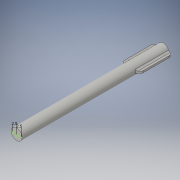
# Autodesk Inventor part: Nathan_Practice_9
Saved by Autodesk Inventor 2016 (Build 200138000, 138)
## iProperties
Created: 2017-03-09
Part Number: Nathan_Practice_9
Material: Generic
Document SubType Name: Modeling
Designer: Student
Density: 1 g/cm^3
Appearance: Default
Author: Student
Autodesk Inventor part; units mm, degrees
ref_plane "YZ Plane" through (0, 0, 0) normal (1, 0, 0) x (0, 1, 0)
ref_plane "XZ Plane" through (0, 0, 0) normal (0, 1, 0) x (-1, 0, 0)
ref_plane "XY Plane" through (0, 0, 0) normal (0, 0, 1) x (1, 0, 0)
sketch "Sketch1" plane through (0, 0, 0) normal (0, 0, 1) x (1, 0, 0)
  circle A0 centre (0, 0) radius 3
  dimension "d0" = 6
  constraints: 1 centre point, 1 coincident
  measures "d0" diameter of A0
extrude "Extrusion1" add sketch "Sketch1" along normal blind 80
sketch "Sketch2" plane through (0, 0, 0) normal (0, 1, 0) x (-1, 0, 0)
  line L0 (-3, 0) -> (3, 0) projected
  line L1 (5, 0) -> (5, 18)
  line L2 (-5, 0) -> (-5, 18)
  line L3 (-3, 0) -> (-3, 80) projected
  line L4 (3, 0) -> (3, 80) projected
  line L5 (5, 18) -> (2, 18)
  line L6 (2, 18) -> (2, 0)
  line L7 (5, 0) -> (2, 0)
  line L8 (-5, 18) -> (-2, 18)
  line L9 (-2, 18) -> (-2, 0)
  line L10 (-2, 0) -> (-5, 0)
  point P0 (0, 0)
  dimension "d3" = 2
  dimension "d4" = 2
  dimension "d6" = 18
  dimension "d9" = 3
  dimension "d10" = 18
  dimension "d11" = 3
  constraints: 16 end point, 3 perpendicular, 2 horizontal, 2 point on line, 2 vertical, 1 collinear
  measures "d3" distance of L0.start L2.start
  measures "d4" distance of L0.end L1.start
  measures "d6" distance of L2.start L2.end
  measures "d9" distance of L1.end L5.end
  measures "d10" distance between parallel lines of L5 L7
  measures "d11" distance of L2.end L8.end
extrude "Extrusion2" add sketch "Sketch2" along normal mid plane 1
fillet "Fillet1" radius 2 4 edges at (5, 0, 18) (-5, 0, 18) (-5, 0, 0) (5, 0, 0)
fillet "Fillet2" radius 1 4 edges at (-2.958, 0.5, 9) (-2.958, -0.5, 9) (2.958, -0.5, 9) (2.958, 0.5, 9)
sketch "Sketch4" plane through (0, 0, 80) normal (0, 0, 1) x (1, 0, 0)
  point P0 (-2.5, 0)
  point P1 (2.5, 0)
  point P2 (0, 0)
  dimension "d24" = 2.5
  dimension "d25" = 2.5
  measures "d24" distance of point (-2.5, 0) point (0, 0)
  measures "d25" distance of point (2.5, 0) point (0, 0)
body "Solid1"
